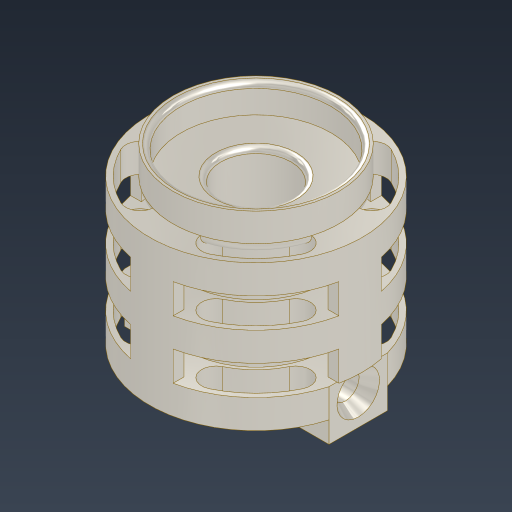
# Autodesk Inventor part: wheel
Saved by Autodesk Inventor 2023 (Build 270158000, 158)
## iProperties
Created: 2025-03-30
Part Number: wheel
Material: ABS Plastic
Document SubType Name: Modeling
Designer: szymo
Density: 0.822506 g/cm^3
Appearance: Titanium
Mass: 10 g
Surface Area: 33.7134 cm^2
Volume: 3.23848 cm^3
Author: szymo
Autodesk Inventor part; units mm, degrees
ref_plane "YZ Plane" through (0, 0, 0) normal (1, 0, 0) x (0, 1, 0)
ref_plane "XZ Plane" through (0, 0, 0) normal (0, 1, 0) x (-1, 0, 0)
ref_plane "XY Plane" through (0, 0, 0) normal (0, 0, 1) x (1, 0, 0)
sketch "Sketch1" plane through (0, 0, 0) normal (0, 1, 0) x (-1, 0, 0)
  circle A0 centre (0, 0) radius 15
  dimension "d0" = 30
  constraints: 1 centre point, 1 coincident
  measures "d0" diameter of A0
extrude "Extrusion1" [suppressed]
sketch "Sketch3" plane through (0, 0, 0) normal (1, 0, 0) x (0, 1, 0)
  line L0 (-1.775, 2.8512) -> (-1.775, -26.1972) projected
  line L1 (4.3, -3) -> (13.7793, -3)
  line L2 (13.9, -10) -> (11.2, -10)
  line L3 (11.2, -10) -> (11.2, -6.8)
  line L4 (11.2, -6.8) -> (8.4125, -6.8)
  line L5 (8.4125, -6.8) -> (8.4125, -10)
  line L6 (8.4125, -10) -> (5.7125, -10)
  line L7 (5.7125, -10) -> (5.7125, -6.8)
  line L8 (5.7125, -6.8) -> (2.925, -6.8)
  line L9 (2.925, -6.8) -> (2.925, -10)
  line L10 (2.925, -10) -> (0.225, -10)
  line L11 (4.3, -3) -> (-1.775, -3)
  line L12 (0.225, -10) -> (0.225, -6.8)
  line L13 (0.225, -6.8) -> (-1.775, -6.8)
  line L14 (-1.775, -6.8) -> (-1.775, -3)
  line L15 (13.7793, -3) -> (13.9, -3)
  line L16 (13.9, -3) -> (13.9, -6.8)
  line L17 (13.9, -6.8) -> (13.9, -6.8)
  line L18 (13.9, -6.8) -> (13.9, -10)
  line L19 (13.9, -6.8) -> (11.2, -6.8) construction
  line L20 (8.4125, -6.8) -> (5.7125, -6.8) construction
  line L21 (2.925, -6.8) -> (0.225, -6.8) construction
  line L22 (-1.775, -3.3) -> (13.9, -3.3)
  line L23 (-1.775, -26.1972) -> (-1.775, -3)
  line L24 (17.2, -15) -> (-0.4918, -15)
  line L25 (16.9387, -10) -> (-0.5866, -10)
  line L26 (-7.9373, 0) -> (24.3062, 0) projected
  arc A0 (-2.9483, -0.5546) -> (-0.4617, -2.9643) centre (0, 0) ccw projected
  line L27 (17.3, -4.0467) -> (17.3, 4.0467)
  line L28 (19.7, 6) -> (19.7, -6)
  line L29 (17.3, -2.7234) -> (17.3, -14.5692)
  line L30 (14.65, 6.3) -> (14.65, -6.3)
  line L31 (13.9, -7.8) -> (16.55, -7.8)
  line L32 (16.55, -7.8) -> (16.55, -7.05)
  line L33 (16.55, -7.05) -> (13.9, -7.05)
  line L34 (14.65, 6.3) -> (14.65, -6.3)
  line L35 (13.9, -7.05) -> (13.9, -6.8)
  point P0 (0, 0)
  point P1 (17.3, 0)
  point P2 (-1.775, -3.3)
  point P3 (-1.775, -6.8)
  point P4 (-1.775, -3.3)
  point P5 (-1.775, -6.8)
  dimension "d6" = 2.7
  dimension "d8" = 2.7
  dimension "d10" = 2.7
  dimension "d14" = 0.3
  dimension "d15" = 3.5
  dimension "d16" = 0
  dimension "d17" = 2
  dimension "d18" = 2.7875
  dimension "d19" = 2.7875
  dimension "d20" = 15
  dimension "d22" = 0
  dimension "d23" = 0
  dimension "d25" = 5
  dimension "d110" = 3.4
  dimension "d116" = 0
  dimension "d117" = 0.75
  dimension "d118" = 0.75
  dimension "d119" = 0.75
  dimension "d120" = 0.75
  constraints: 68 end point, 16 perpendicular, 7 horizontal, 7 vertical, 6 point on line, 4 collinear, 1 midpoint, 6 other
  measures "d6" distance of L2.start L2.end
  measures "d8" distance of L5.end L6.end
  measures "d10" distance of L9.end L10.end
  measures "d14" distance between parallel lines of L15 L22
  measures "d15" distance between parallel lines of L17 L22
  measures "d16" distance between parallel lines of L16 L18
  measures "d17" distance between parallel lines of L12 L14
  measures "d18" distance between parallel lines of L3 L5
  measures "d19" distance between parallel lines of L9 L7
  measures "d20" distance from line of L24 point (17.3, 0)
  measures "d22" distance between parallel lines of L25 L2
  measures "d23" distance between parallel lines of L25 L6
  measures "d25" distance between parallel lines of L24 L25
  measures "d110" distance between parallel lines of L16 L27
  measures "d116" distance between parallel lines of L27 L29
  measures "d117" distance between parallel lines of L16 L30
  measures "d118" distance from line of L33 L30.end
  measures "d119" distance between parallel lines of L31 L33
  measures "d120" distance between parallel lines of L32 L29
revolve "Revolution1" add sketch "Sketch3" angle 360 about axis through (0, -10, 0) along (0, 1, 0) contours L22 L16 L18 L2 L3 L4 L5 L6 L7 L8 L9 L10 L12 L13 L0 | L33 L32 L31 L18
sketch "Sketch4" plane through (0, -1.775, 0) normal (0, -1, 0) x (1, 0, 0)
  circle A0 centre (0, 0) radius 10 projected
  circle A1 centre (0, 0) radius 6.8 projected
  line L0 (-9.6144, -2.75) -> (-6.2191, -2.75)
  line L1 (-6.2191, -2.75) -> (-6.2191, 2.75)
  line L2 (-6.2191, 2.75) -> (-9.6144, 2.75)
  line L3 (-9.6144, 2.75) -> (-9.6144, -2.75)
  line L4 (5.9998, -2.75) -> (9.6144, -2.75)
  line L5 (9.6144, -2.75) -> (9.6144, 2.75)
  line L6 (9.6144, 2.75) -> (5.9998, 2.75)
  line L7 (5.9998, 2.75) -> (5.9998, -2.75)
  circle A2 centre (0, 0) radius 10 projected
  line L8 (-10, 0) -> (10, 0) construction
  circle A3 centre (0, 0) radius 6.6 projected
  point P0 (9.6144, 2.75)
  point P1 (6.2191, 2.75)
  point P2 (6.2191, -2.75)
  point P3 (9.6144, -2.75)
  point P4 (-9.6144, 2.75)
  point P5 (-9.6144, -2.75)
  dimension "d26" = 5.5
  dimension "d28" = 5.5
  dimension "d30" = 2.75
  dimension "d31" = 2.75
  dimension "d32" = 2.75
  dimension "d33" = 2.75
  constraints: 18 end point, 4 parallel, 4 point on circle, 3 perpendicular, 2 horizontal, 1 coincident, 1 midpoint, 4 other
  measures "d26" distance of L1.end L0.end
  measures "d28" distance of L5.end L4.end
  measures "d30" distance from line of L0.end L8
  measures "d31" distance between parallel lines of L2 L8
  measures "d32" distance between parallel lines of L4 L8
  measures "d33" distance between parallel lines of L8 L6
extrude "Extrusion2" add sketch "Sketch4" against normal up to surface (4.7 mm away) contours L5 L4 A1 L6 | L2 A1 L0 L3
sketch "Sketch5" plane through (6.2191, -1.775, -2.75) normal (0, -1, 0) x (1, 0, 0)
  circle A0 centre (-5.9998, 2.75) radius 6.6 projected
  circle A1 centre (-5.9998, 2.75) radius 3.1 projected
  arc A2 (0, 5.5) -> (-12.4382, 5.5) centre (-6.2191, 2.75) ccw projected
  arc A3 (3.3953, 5.5) -> (-15.8336, 5.5) centre (-6.2191, 2.75) ccw projected
  arc A4 (-15.8336, 5.5) -> (-15.8336, 0) centre (-6.2191, 2.75) ccw projected
  arc A5 (-15.8336, 0) -> (3.3953, 0) centre (-6.2191, 2.75) ccw projected
  arc A6 (-12.4382, 0) -> (0, 0) centre (-6.2191, 2.75) ccw projected
  arc A7 (3.3953, 0) -> (3.3953, 5.5) centre (-6.2191, 2.75) ccw projected
  line L0 (3.3953, 5.5) -> (3.3953, 0) projected
  line L1 (3.3953, 0) -> (0, 0) projected
  line L2 (-12.4382, 0) -> (-15.8336, 0) projected
  line L3 (-15.8336, 0) -> (-15.8336, 5.5) projected
  line L4 (0, 5.5) -> (3.3953, 5.5) projected
  line L5 (-15.8336, 5.5) -> (-12.4382, 5.5) projected
extrude "Extrusion3" cut sketch "Sketch5" against normal up to surface (4.7 mm away) contours A7 L0 | L3 A4
fillet "Fillet1" radius 0.5 3 edges at (0, 16.55, 7.05) (0, 13.9, 3.3) (0, -1.775, 3.3)
sketch "Sketch8" plane through (9.6144, -1.775, 2.75) normal (1, 0, 0) x (0, 0, -1)
  line L0 (0, 0) -> (0, 2) projected
  line L1 (5.5, 0) -> (0, 0) projected
  line L2 (5.5, 0) -> (5.5, 2) projected
  line L3 (5.5, 4.7) -> (0, 4.7) projected
  line L4 (5.5, 4.7) -> (5.5, 2) projected
  line L5 (0, 4.7) -> (5.5, 4.7) projected
  line L6 (0, 2) -> (0, 4.7) projected
  line L7 (0, 4.7) -> (5.5, 1)
  line L8 (5.5, 4.7) -> (0, 1)
  line L9 (0, 0) -> (0, 2) projected
  line L10 (0, 1) -> (5.5, 1)
  point P0 (2.75, 1.775)
  point P1 (2.75, 2.85)
  dimension "d130" = 1
  constraints: 6 end point, 3 midpoint, 1 horizontal
  measures "d130" distance between parallel lines of L1 L10
sketch "Sketch9" plane through (-9.6144, -1.775, -2.75) normal (-1, 0, 0) x (0, 0, 1)
  line L0 (0, 0) -> (0, 2) projected
  line L1 (5.5, 0) -> (0, 0) projected
  line L2 (5.5, 0) -> (5.5, 2) projected
  line L3 (9.35, 0) -> (5.5, 0) projected
  line L4 (5.5, 4.7) -> (5.5, 2) projected
  line L5 (0, 4.7) -> (5.5, 4.7) projected
  line L6 (0, 2) -> (0, 4.7) projected
  line L7 (5.5, 4.7) -> (0, 1)
  line L8 (0, 4.7) -> (5.5, 1)
  line L9 (0, 1) -> (5.5, 1)
  point P0 (2.75, 1.775)
  point P1 (2.75, 2.85)
  dimension "d129" = 1
  constraints: 6 end point, 3 midpoint, 1 horizontal
  measures "d129" distance between parallel lines of L9 L1
hole "Hole3" at (-9.6144, 1.075, 0) direction (1, 0, 0) diameter 2.6 depth 8.8 countersink diameter 4 countersink angle 60
hole "Hole4" at (9.6144, 1.075, 0) direction (-1, 0, 0) diameter 2.6 depth 8.8 countersink diameter 4 countersink angle 60
ref_plane "Work Plane4" through (2.75, 17.2, 9.6144) normal (0, 1, 0) x (1, 0, 0)
sketch "Sketch12" plane through (2.75, 13.9, 9.6144) normal (0, 1, 0) x (1, 0, 0)
  circle A0 centre (-10.9, 9.6144) radius 1.35 construction
  circle A1 centre (-2.75, 9.6144) radius 6.8 projected
  circle A2 centre (-2.75, 9.6144) radius 10 projected
  line L0 (-2.75, 9.6144) -> (-12.75, 9.6144)
  circle A3 centre (-2.75, 9.6144) radius 10 projected
  circle A4 centre (-2.75, 9.6144) radius 6.8 projected
  circle A5 centre (-2.75, 9.6144) radius 8.15 construction
  arc A6 (-11.7552, 7.327) -> (-9.4889, 7.9027) centre (-10.7882, 8.2691) ccw construction
  circle A7 centre (-10.7882, 10.9598) radius 1.35 construction
  circle A8 centre (-2.75, 9.6144) radius 6.8
  circle A9 centre (-2.75, 9.6144) radius 9.5
  arc A10 (-11.7323, 6.521) -> (-9.1794, 7.4002) centre (-10.4558, 6.9606) ccw
  arc A11 (-9.1794, 11.8287) -> (-11.7323, 12.7078) centre (-10.4558, 12.2683) ccw
  arc A12 (-11.7552, 7.327) -> (-11.7323, 6.521) centre (-10.4558, 6.9606) ccw construction
  arc A13 (-12.1197, 8.0462) -> (-11.7552, 7.327) centre (-10.7882, 8.2691) ccw construction
  arc A14 (-9.4889, 7.9027) -> (-11.7552, 7.327) centre (-10.4558, 6.9606) ccw construction
  arc A15 (-9.1794, 7.4002) -> (-9.4889, 7.9027) centre (-10.4558, 6.9606) ccw construction
  arc A16 (-9.4889, 7.9027) -> (-9.4567, 8.4919) centre (-10.7882, 8.2691) ccw construction
  arc A17 (-9.4567, 8.4919) -> (-12.1197, 8.0462) centre (-10.7882, 8.2691) ccw construction
  arc A18 (-9.4889, 11.3262) -> (-9.1794, 11.8287) centre (-10.4558, 12.2683) ccw construction
  arc A19 (-11.7552, 11.9019) -> (-9.4889, 11.3262) centre (-10.4558, 12.2683) ccw construction
  arc A20 (-11.7323, 12.7078) -> (-11.7552, 11.9019) centre (-10.4558, 12.2683) ccw construction
  arc A21 (-6.9141, 1.0757) -> (-5.7306, 3.5025) centre (-6.3223, 2.2891) ccw
  arc A22 (-8.862, 6.6339) -> (-11.2888, 5.4504) centre (-10.0754, 6.0421) ccw
  arc A23 (0.3434, 0.6322) -> (-0.5358, 3.185) centre (-0.0962, 1.9086) ccw
  arc A24 (-4.9642, 3.185) -> (-5.8434, 0.6322) centre (-5.4038, 1.9086) ccw
  arc A25 (5.7888, 5.4504) -> (3.362, 6.6339) centre (4.5754, 6.0421) ccw
  arc A26 (0.2306, 3.5025) -> (1.4141, 1.0757) centre (0.8223, 2.2891) ccw
  arc A27 (6.2323, 12.7078) -> (3.6794, 11.8287) centre (4.9558, 12.2683) ccw
  arc A28 (3.6794, 7.4002) -> (6.2323, 6.521) centre (4.9558, 6.9606) ccw
  arc A29 (1.4141, 18.1532) -> (0.2306, 15.7264) centre (0.8223, 16.9398) ccw
  arc A30 (3.362, 12.595) -> (5.7888, 13.7785) centre (4.5754, 13.1868) ccw
  arc A31 (-5.8434, 18.5967) -> (-4.9642, 16.0438) centre (-5.4038, 17.3203) ccw
  arc A32 (-0.5358, 16.0438) -> (0.3434, 18.5967) centre (-0.0962, 17.3203) ccw
  arc A33 (-11.2888, 13.7785) -> (-8.862, 12.595) centre (-10.0754, 13.1868) ccw
  arc A34 (-5.7306, 15.7264) -> (-6.9141, 18.1532) centre (-6.3223, 16.9398) ccw
  point P0 (-2.8936, 9.6144)
  point P1 (-9.55, 9.6144)
  point P2 (-9.55, 9.6144)
  point P3 (-12.25, 9.6144)
  point P4 (-12.25, 9.6144)
  point P5 (-5.7306, 15.7264)
  point P6 (-5.3827, 15.9704)
  point P7 (-6.3434, 18.2896)
  point P8 (-6.9141, 18.1532)
  point P9 (-11.2888, 13.7785)
  point P10 (-11.4252, 13.2078)
  point P11 (-9.106, 12.2472)
  point P12 (0.8434, 18.2896)
  point P13 (-0.1173, 15.9704)
  point P14 (0.2306, 15.7264)
  point P15 (3.362, 12.595)
  point P16 (3.606, 12.2472)
  point P17 (5.9252, 13.2078)
  point P18 (5.7888, 13.7785)
  point P19 (1.4141, 18.1532)
  point P20 (5.9252, 6.0211)
  point P21 (3.606, 6.9817)
  point P22 (3.362, 6.6339)
  point P23 (0.2306, 3.5025)
  point P24 (-0.1173, 3.2584)
  point P25 (0.8434, 0.9392)
  point P26 (1.4141, 1.0757)
  point P27 (5.7888, 5.4504)
  point P28 (-6.3434, 0.9392)
  point P29 (-5.3827, 3.2584)
  point P30 (-5.7306, 3.5025)
  point P31 (-8.862, 6.6339)
  point P32 (-9.106, 6.9817)
  point P33 (-11.4252, 6.0211)
  point P34 (-11.2888, 5.4504)
  point P35 (-6.9141, 1.0757)
  dimension "d131" = 0
  dimension "d132" = 0.5
  dimension "d133" = 2.7
  dimension "d136" = 360
  constraints: 72 point on circle, 31 centre point, 4 coincident, 4 equal radius, 4 point on line, 2 end point, 2 horizontal alignment, 2 tangent, 1 horizontal, 67 other
  measures "d131" distance of A0.start point (-9.55, 9.614)
  measures "d132" distance of point (-12.25, 9.614) L0.end
  measures "d133" diameter of A0
extrude "Extrusion6" cut sketch "Sketch12" against normal up to surface (13.675 mm away) contours A1 A29 A32 A9 A30 A27 | A27 A30 | A25 A28 A9 A26 A23 A1 | A25 A28 | A29 A32 | A23 A26 | A1 A33 A11 A9 A34 A31 | A31 A34 | A21 A24 A9 A22 A10 A1 | A21 A24 | A33 A11 | A10 A22
sketch "Sketch17" plane through (0, 13.9, 0) normal (0, 1, 0) x (1, 0, 0)
  circle A0 centre (0, 0) radius 7.8 projected
  circle A1 centre (0, 0) radius 3.8 projected
extrude "Extrusion9" add sketch "Sketch17" against normal blind 1
fillet "Fillet7" radius 1 4 edges at (-5.5154, 12.9, 5.5154) (5.5154, 12.9, 5.5154) (5.5154, 12.9, -5.5154) (-5.5154, 12.9, -5.5154)
sketch "Sketch13" plane through (0, 13.9, 0) normal (0, 1, 0) x (0, 0, -1)
  circle A0 centre (0, 0) radius 8.8
  line L0 (-6.4992, -2) -> (-9.798, -2)
  arc A1 (10, 0) -> (10, 0) centre (0, 0) ccw projected
  line L1 (-9.798, 2) -> (-6.4992, 2)
  line L2 (-9.2378, 0) -> (9.2378, 0)
  arc A2 (6.112, -2.9806) -> (6.112, 2.9806) centre (0, 0) ccw projected
  line L3 (6.4992, -2) -> (9.798, -2)
  line L4 (9.798, 2) -> (6.4992, 2)
  circle A3 centre (0, 0) radius 6.8
  circle A4 centre (0, 0) radius 10 projected
  line L5 (0, 10) -> (0, -10)
  line L6 (2, -9.798) -> (2, 9.798)
  line L7 (-2, 9.798) -> (-2, -9.798)
  arc A5 (2.75, -6.2191) -> (2.75, 6.2191) centre (0, 0) ccw projected
  point P0 (-2.75, 5.9998)
  point P1 (-2.75, -5.9998)
  point P2 (2.75, 5.9998)
  point P3 (2.75, -5.9998)
  point P4 (-8.5697, -2)
  point P5 (-2, 8.5697)
  point P6 (2, 8.5697)
  point P7 (-2, -8.5697)
  point P8 (2, -8.5697)
  point P9 (-1.5, 6.6325)
  point P10 (1.5, 6.6325)
  point P11 (8.5697, -2)
  point P12 (8.5697, 2)
  point P13 (1.5, -6.6325)
  point P14 (-1.5, -6.6325)
  point P15 (-6.6325, -1.5)
  point P16 (-6.6325, 1.5)
  point P17 (6.6325, -1.5)
  point P18 (2, 6.4992)
  point P19 (-2, 6.4992)
  point P20 (2, -6.4992)
  point P21 (-2, -6.4992)
  dimension "d87" = 2
  dimension "d88" = 2
  dimension "d89" = 2
  dimension "d90" = 2
  dimension "d93" = 2
  dimension "d114" = 2
  dimension "d115" = 2
  constraints: 16 end point, 6 parallel, 4 midpoint, 4 point on circle, 2 coincident, 1 centre point, 1 concentric, 1 horizontal, 1 vertical, 15 other
  measures "d87" distance between parallel lines of L0 L2
  measures "d88" distance between parallel lines of L1 L2
  measures "d89" distance between parallel lines of L3 L2
  measures "d90" distance between parallel lines of L4 L2
  measures "d114" distance between parallel lines of L7 L5
  measures "d115" distance between parallel lines of L6 L5
extrude "Extrusion7" add sketch "Sketch13" against normal up to surface (10.975 mm away) contours L2 A2 L4 A0 | A0 L4 A1 L3 | A0 L3 A2 L2 | L6 A3 L5 A0 | A0 L5 A1 L6 | L6 A1 L5 A0 | A0 L5 A3 L6 | L5 A3 L7 A0 | A0 L7 A1 L5 | L5 A1 L7 A0 | A0 L7 A3 L5 | L1 A3 L2 A0 | A0 L0 A1 L1 | A0 L2 A3 L0
sketch "Sketch18" plane through (0, 0, 0) normal (1, 0, 0) x (0, 1, 0)
  line L0 (-5.44, 0) -> (20.215, 0) projected
  line L1 (13.9, -10) -> (13.9, 10) projected
  line L2 (2.925, 6.4992) -> (2.925, 9.798) projected
  line L3 (5.7125, 9.798) -> (5.7125, 6.4992) projected
  line L4 (8.4125, 6.4992) -> (8.4125, 9.798) projected
  line L5 (11.2, 9.798) -> (11.2, 6.4992) projected
  line L6 (13.9, 10) -> (2.925, 10)
  line L7 (0.225, 10) -> (13.9, 10) projected
  line L8 (2.925, 9.798) -> (2.925, 10)
  line L9 (5.7125, 9.798) -> (5.7125, 10)
  line L10 (8.4125, 9.798) -> (8.4125, 10)
  line L11 (11.2, 9.798) -> (11.2, 10)
  line L12 (2.925, 9) -> (5.7125, 9)
  line L13 (5.7125, 6.4992) -> (5.7125, 9.798) projected
  line L14 (2.925, 6.4992) -> (5.7125, 6.4992)
  line L15 (8.4125, 6.4992) -> (11.2, 6.4992) projected
  line L16 (8.4125, 6.4992) -> (11.2, 6.4992)
  line L17 (8.4125, 9.798) -> (8.4125, 6.4992) projected
  line L18 (8.4125, 9) -> (11.2, 9)
  point P0 (0, 0)
  dimension "d141" = 1
  dimension "d142" = 1
  constraints: 18 end point, 8 point on line, 6 perpendicular, 1 collinear, 1 vertical
  measures "d141" distance between parallel lines of L7 L12
  measures "d142" distance between parallel lines of L18 L7
revolve "Revolution4" cut sketch "Sketch18" angle 360 about axis through (0, -10, 0) along (0, 1, 0) contours L2 L12 L3 L14 | L4 L18 L5 L15
equation "\"d18\" = d19"
equation "\"d30\" = d31"
equation "\"d32\" = d33"
equation "\"d88\" = d87"
equation "\"d89\" = d87"
equation "\"d90\" = d87"
body "Solid1"
